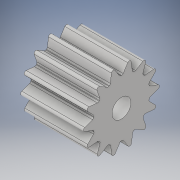
# Autodesk Inventor part: 30_Cube_Z_Focus_MGN12_manual_gear_v3
Saved by Autodesk Inventor 2019 (Build 230136000, 136)
## iProperties
Created: 2021-05-14
Part Number: 30_Cube_Z_Focus_MGN12_manual_gear_v3
Material: Generic
Document SubType Name: Modeling
Designer: diederichbenedict
Density: 1 g/cm^3
Appearance: Default
Author: diederichbenedict
Autodesk Inventor part; units mm, degrees
ref_plane "YZ Plane" through (0, 0, 0) normal (1, 0, 0) x (0, 1, 0)
ref_plane "Work Plane1" through (-11.1225, -8.6007, 24.2188) normal (-1, 0, 0) x (0, 0, 1)
sketch "Sketch1" plane through (-11.1225, -8.6007, 24.2188) normal (-1, 0, 0) x (0, 0, 1)
  line L0 (-16.0994, 9.698) -> (-17.9787, 9.014) projected
  line L1 (-17.9787, 9.014) -> (-17.9787, 8.614) projected
  line L2 (-17.9787, 8.614) -> (-16.0994, 7.9299) projected
  line L3 (-16.0994, 9.698) -> (-16.0994, 7.9299) projected
  circle A0 centre (-22.4787, 8.6007) radius 4.5
  line L4 (-17.9787, 8.6007) -> (-16.347, 8.6007)
  line L5 (-16.347, 8.6007) -> (-16.347, 8.7507)
  line L6 (-16.347, 8.7507) -> (-18.0447, 9.3686)
  line L7 (-16.347, 8.6007) -> (-16.347, 8.4007)
  line L8 (-16.347, 8.6007) -> (-16.147, 8.6007) construction
  line L9 (-16.347, 8.4007) -> (-18.0543, 7.7793)
  line L10 (-29.1546, 8.6007) -> (-13.9235, 8.6007) projected
  point P0 (-24.2188, 8.6007)
  dimension "d0" = 0.15
  dimension "d1" = 110
  dimension "d2" = 0.2
  dimension "d3" = 90
  dimension "a1" = 110
  dimension "d23" = 9
  constraints: 12 end point, 3 point on circle, 2 horizontal, 2 perpendicular, 2 point on line, 1 centre point, 1 tangent, 1 vertical
  measures "d0" distance of L4.end L5.end
  measures "d1" angle of L5 L6
  measures "d2" distance of L4.end L7.end
  measures "d3" angle of L7 L8
  measures "a1" angle of L7 L9
  measures "d23" diameter of A0
extrude "Extrusion1" add sketch "Sketch1" along normal mid plane 10 contours L6 L5 L4 L2 L1 L0 | L0 L1 A0 L6 | A0 L10 | L7 L9 L2 L4 | L2 L4 A0 | L10 A0 | L9 A0 L4 L2
fillet "Fillet1" radius 0.3 4 edges at (-11.1225, 0.7679, 6.174) (-11.1225, 0.15, 7.8718) (-11.1225, -0.2, 7.8718) (-11.1225, -0.8214, 6.1644)
pattern_circular "Circular Pattern2" count 14 over 360 about axis through (-11.1225, 0, 1.7401) along (-1, 0, 0) of "Extrusion1", "Fillet1"
ref_plane "Work Plane2" through (-11.1225, -8.6007, 24.2188) normal (1, 0, 0) x (0, 0, -1)
sketch "Sketch2" plane through (-6.1225, -8.6007, 24.2188) normal (1, 0, 0) x (0, 0, -1)
  arc A0 (17.8849, 9.3104) -> (18.0758, 9.5304) centre (17.7823, 9.5924) ccw projected
  line L0 (17.8849, 9.3104) -> (16.6407, 8.8576) projected
  arc A1 (16.6407, 8.8576) -> (16.6407, 8.2938) centre (16.7433, 8.5757) ccw projected
  line L1 (16.6407, 8.2938) -> (17.8967, 7.8366) projected
  arc A2 (18.0869, 7.6201) -> (17.8967, 7.8366) centre (17.7941, 7.5547) ccw projected
  arc A3 (20.7646, 4.28) -> (20.5926, 4.515) centre (20.4669, 4.2427) ccw projected
  line L2 (20.7646, 4.28) -> (20.9292, 2.9662) projected
  arc A4 (20.9292, 2.9662) -> (21.4789, 2.8407) centre (21.2269, 3.0035) ccw projected
  line L3 (21.4789, 2.8407) -> (22.204, 3.9635) projected
  arc A5 (22.4575, 4.1007) -> (22.204, 3.9635) centre (22.456, 3.8007) ccw projected
  arc A6 (22.809, 3.9641) -> (22.5521, 4.1013) centre (22.557, 3.8013) ccw projected
  line L4 (22.809, 3.9641) -> (23.5274, 2.8519) projected
  arc A7 (23.5274, 2.8519) -> (24.077, 2.9773) centre (23.7794, 3.0146) ccw projected
  line L5 (24.077, 2.9773) -> (24.2432, 4.3035) projected
  arc A8 (24.412, 4.5371) -> (24.2432, 4.3035) centre (24.5409, 4.2662) ccw projected
  arc A9 (24.788, 4.5666) -> (24.4971, 4.5787) centre (24.6316, 4.3106) ccw projected
  line L6 (24.788, 4.5666) -> (25.9178, 3.8762) projected
  arc A10 (25.9178, 3.8762) -> (26.3586, 4.2277) centre (26.0743, 4.1321) ccw projected
  line L7 (26.3586, 4.2277) -> (25.933, 5.4947) projected
  arc A11 (25.9837, 5.7784) -> (25.933, 5.4947) centre (26.2173, 5.5902) ccw projected
  arc A12 (26.3097, 5.968) -> (26.0423, 5.8527) centre (26.2798, 5.6695) ccw projected
  line L8 (26.3097, 5.968) -> (27.6272, 5.8362) projected
  arc A13 (27.6272, 5.8362) -> (27.8718, 6.3442) centre (27.657, 6.1347) ccw projected
  line L9 (27.8718, 6.3442) -> (26.9385, 7.301) projected
  arc A14 (26.8611, 7.5786) -> (26.9385, 7.301) centre (27.1533, 7.5105) ccw projected
  arc A15 (27.0726, 7.8909) -> (26.8817, 7.671) centre (27.1752, 7.609) ccw projected
  line L10 (27.0726, 7.8909) -> (28.3168, 8.3438) projected
  arc A16 (28.3168, 8.3438) -> (28.3168, 8.9076) centre (28.2142, 8.6257) ccw projected
  line L11 (28.3168, 8.9076) -> (27.0608, 9.3647) projected
  arc A17 (26.8706, 9.5813) -> (27.0608, 9.3647) centre (27.1634, 9.6466) ccw projected
  arc A18 (26.9256, 9.9544) -> (26.849, 9.6734) centre (27.1404, 9.7449) ccw projected
  line L12 (26.9256, 9.9544) -> (27.8501, 10.9022) projected
  arc A19 (27.8501, 10.9022) -> (27.6055, 11.4102) centre (27.6353, 11.1117) ccw projected
  line L13 (27.6055, 11.4102) -> (26.2755, 11.2771) projected
  arc A20 (26.0102, 11.3897) -> (26.2755, 11.2771) centre (26.2456, 11.5757) ccw projected
  arc A21 (25.8979, 11.7498) -> (25.9508, 11.4634) centre (26.1822, 11.6542) ccw projected
  line L14 (25.8979, 11.7498) -> (26.3195, 13.0049) projected
  arc A22 (26.3195, 13.0049) -> (25.8787, 13.3564) centre (26.0352, 13.1004) ccw projected
  line L15 (25.8787, 13.3564) -> (24.7382, 12.6595) projected
  arc A23 (24.4504, 12.6458) -> (24.7382, 12.6595) centre (24.5818, 12.9154) ccw projected
  arc A24 (24.1929, 12.9214) -> (24.3649, 12.6863) centre (24.4906, 12.9587) ccw projected
  line L16 (24.1929, 12.9214) -> (24.0283, 14.2352) projected
  arc A25 (24.0283, 14.2352) -> (23.4786, 14.3606) centre (23.7306, 14.1979) ccw projected
  line L17 (23.4786, 14.3606) -> (22.7535, 13.2379) projected
  arc A26 (22.5, 13.1006) -> (22.7535, 13.2379) centre (22.5014, 13.4006) ccw projected
  arc A27 (22.1485, 13.2373) -> (22.4054, 13.1001) centre (22.4005, 13.4001) ccw projected
  line L18 (22.1485, 13.2373) -> (21.4301, 14.3495) projected
  arc A28 (21.4301, 14.3495) -> (20.8804, 14.2241) centre (21.1781, 14.1867) ccw projected
  line L19 (20.8804, 14.2241) -> (20.7142, 12.8978) projected
  arc A29 (20.5455, 12.6642) -> (20.7142, 12.8978) centre (20.4166, 12.9351) ccw projected
  arc A30 (20.1694, 12.6348) -> (20.4604, 12.6227) centre (20.3259, 12.8908) ccw projected
  line L20 (20.1694, 12.6348) -> (19.0396, 13.3252) projected
  arc A31 (19.0396, 13.3252) -> (18.5988, 12.9737) centre (18.8832, 13.0692) ccw projected
  line L21 (18.5988, 12.9737) -> (19.0245, 11.7067) projected
  arc A32 (18.9738, 11.423) -> (19.0245, 11.7067) centre (18.7401, 11.6112) ccw projected
  arc A33 (18.6478, 11.2333) -> (18.9152, 11.3487) centre (18.6777, 11.5319) ccw projected
  line L22 (18.6478, 11.2333) -> (17.3303, 11.3652) projected
  arc A34 (17.3303, 11.3652) -> (17.0857, 10.8572) centre (17.3005, 11.0667) ccw projected
  line L23 (17.0857, 10.8572) -> (18.019, 9.9004) projected
  arc A35 (18.0963, 9.6228) -> (18.019, 9.9004) centre (17.8042, 9.6909) ccw projected
  circle A36 centre (22.4787, 8.6007) radius 1.5
  arc A37 (18.0319, 7.247) -> (18.1085, 7.528) centre (17.8171, 7.4564) ccw projected
  line L24 (18.0319, 7.247) -> (17.1074, 6.2991) projected
  arc A38 (17.1074, 6.2991) -> (17.352, 5.7912) centre (17.3222, 6.0897) ccw projected
  line L25 (17.352, 5.7912) -> (18.682, 5.9242) projected
  arc A39 (18.9473, 5.8117) -> (18.682, 5.9242) centre (18.7118, 5.6257) ccw projected
  arc A40 (19.0596, 5.4516) -> (19.0067, 5.738) centre (18.7752, 5.5472) ccw projected
  line L26 (19.0596, 5.4516) -> (18.6379, 4.1965) projected
  arc A41 (18.6379, 4.1965) -> (19.0787, 3.845) centre (18.9223, 4.101) ccw projected
  line L27 (19.0787, 3.845) -> (20.2192, 4.5419) projected
  arc A42 (20.5071, 4.5556) -> (20.2192, 4.5419) centre (20.3757, 4.2859) ccw projected
  circle A43 centre (22.4787, 8.6007) radius 5.7355 construction
  arc A44 (18.0869, 7.6201) -> (18.1085, 7.528) centre (22.4787, 8.6007) ccw projected
  arc A45 (18.9473, 5.8117) -> (19.0067, 5.738) centre (22.4787, 8.6007) ccw projected
  arc A46 (20.5071, 4.5556) -> (20.5926, 4.515) centre (22.4787, 8.6007) ccw projected
  arc A47 (22.4575, 4.1007) -> (22.5521, 4.1013) centre (22.4787, 8.6007) ccw projected
  arc A48 (24.412, 4.5371) -> (24.4971, 4.5787) centre (22.4787, 8.6007) ccw projected
  arc A49 (25.9837, 5.7784) -> (26.0423, 5.8527) centre (22.4787, 8.6007) ccw projected
  arc A50 (26.8611, 7.5786) -> (26.8817, 7.671) centre (22.4787, 8.6007) ccw projected
  arc A51 (26.8706, 9.5813) -> (26.849, 9.6734) centre (22.4787, 8.6007) ccw projected
  arc A52 (26.0102, 11.3897) -> (25.9508, 11.4634) centre (22.4787, 8.6007) ccw projected
  arc A53 (24.4504, 12.6458) -> (24.3649, 12.6863) centre (22.4787, 8.6007) ccw projected
  arc A54 (22.5, 13.1006) -> (22.4054, 13.1001) centre (22.4787, 8.6007) ccw projected
  arc A55 (20.5455, 12.6642) -> (20.4604, 12.6227) centre (22.4787, 8.6007) ccw projected
  arc A56 (18.9738, 11.423) -> (18.9152, 11.3487) centre (22.4787, 8.6007) ccw projected
  arc A57 (18.0963, 9.6228) -> (18.0758, 9.5304) centre (22.4787, 8.6007) ccw projected
  point P0 (18.2571, 4.7183)
  dimension "d14" = 3
  constraints: 3 point on circle, 2 centre point, 1 coincident
  measures "d14" diameter of A36
extrude "Extrusion2" cut sketch "Sketch2" against normal through all contours A36
sketch "Sketch4" plane through (-11.1225, -8.6007, 24.2188) normal (1, 0, 0) x (0, 0, -1)
  circle A0 centre (22.4787, 8.6007) radius 1.5 projected
  line L0 (50.3605, 10.4929) -> (23.9787, 10.4929)
  line L1 (23.9787, 10.4929) -> (23.9787, 6.4929)
  line L2 (23.9787, 6.4929) -> (50.3605, 6.4929)
  line L3 (50.3605, 6.4929) -> (50.3605, 10.4929)
  line L4 (50.3605, 10.4929) -> (23.9787, 6.4929) construction
  line L5 (23.9787, 10.4929) -> (50.3605, 6.4929) construction
  circle A1 centre (52.5846, 8.8043) radius 4.4101
  circle A2 centre (22.4787, 8.6007) radius 1.5 projected
  point P0 (24.2188, 8.6007)
  point P1 (37.1696, 8.4929)
  dimension "d20" = 4
  constraints: 12 end point, 2 midpoint, 2 parallel, 1 centre point, 1 horizontal, 1 perpendicular, 1 tangent
  measures "d20" distance of L1.end L0.end
extrude "Extrusion3" [suppressed]
equation "\"d1\" = a1"
body "Solid1"
